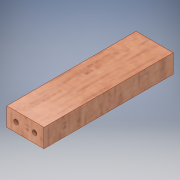
# Autodesk Inventor part: Sensor_Halterung_Drehplatte
Saved by Autodesk Inventor 2018 (Build 220112000, 112)
## iProperties
Created: 2018-03-26
Part Number: Sensor_Halterung_Drehplatte
Material: Holz (Eiche)
Document SubType Name: Modeling
Designer: Julian
Density: 0.76 g/cm^3
Appearance: Weißeiche - natur - mittlerer Glanz
Author: Julian
Autodesk Inventor part; units mm, degrees
ref_plane "YZ Plane" through (0, 0, 0) normal (1, 0, 0) x (0, 1, 0)
ref_plane "XZ Plane" through (0, 0, 0) normal (0, 1, 0) x (-1, 0, 0)
ref_plane "XY Plane" through (0, 0, 0) normal (0, 0, 1) x (1, 0, 0)
sketch "Skizze1" plane through (0, 0, 0) normal (0, 0, 1) x (1, 0, 0)
  line L0 (0, 0) -> (20, 0)
  line L1 (20, 0) -> (20, 69.5)
  line L2 (20, 69.5) -> (0, 69.5)
  line L3 (0, 69.5) -> (0, 0)
  dimension "d0" = 20
  dimension "d1" = 69.5
  constraints: 8 end point, 2 parallel, 1 horizontal, 1 perpendicular
  measures "d0" distance of L2.end L1.end
  measures "d1" distance of L1.end L0.end
extrude "Extrusion1" add sketch "Skizze1" along normal blind 10
sketch "Skizze2" plane through (0, 69.5, 0) normal (0, 1, 0) x (1, 0, 0)
  line L0 (20, 0) -> (20, -10) projected
  line L1 (20, -10) -> (20, -5)
  line L2 (20, -5) -> (17.75, -5)
  line L3 (17.75, -5) -> (2.25, -5)
  point P0 (0, 0)
  dimension "d4" = 2.25
  dimension "d5" = 15.5
  constraints: 6 end point, 1 midpoint, 1 perpendicular, 1 point on line
  measures "d4" distance of L1.end L2.end
  measures "d5" distance of L2.end L3.end
hole "Bohrung1" at (2.25, 69.5, 5) at (17.75, 69.5, 5) direction (0, -1, 0) diameter 2 depth 8 tip angle 118
sketch "Skizze3" plane through (0, 0, 0) normal (0, -1, 0) x (1, 0, 0)
  line L0 (20, 10) -> (0, 10) projected
  line L1 (0, 10) -> (0, 5)
  line L2 (0, 0) -> (0, 10) projected
  line L3 (0, 5) -> (5, 5)
  line L4 (5, 5) -> (15, 5)
  dimension "d13" = 5
  dimension "d14" = 10
  constraints: 6 end point, 1 midpoint, 1 perpendicular, 1 point on line
  measures "d13" distance of L1.end L3.end
  measures "d14" distance of L3.end L4.end
hole "Bohrung2" at (5, 0, 5) at (15, 0, 5) direction (0, 1, 0) diameter 2.5 depth 8 tip angle 118
